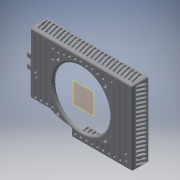
# Autodesk Inventor part: PCB_Cover
Saved by Autodesk Inventor 2019.3 (Build 233278000, 278)
## iProperties
Created: 2020-10-08
Part Number: PCB_Cover
Material: Generisch
Document SubType Name: Modeling
Designer: Nicolas Frick
Density: 1 g/cm^3
Appearance: Vorgabe
Author: Nicolas Frick
Autodesk Inventor part; units mm, degrees
(part 1 of 2)
ref_plane "YZ Plane" through (0, 0, 0) normal (1, 0, 0) x (0, 1, 0)
ref_plane "XZ Plane" through (0, 0, 0) normal (0, 1, 0) x (-1, 0, 0)
ref_plane "XY Plane" through (0, 0, 0) normal (0, 0, 1) x (1, 0, 0)
sketch "Skizze1" plane through (0, 0, 0) normal (0, 0, 1) x (1, 0, 0)
  circle A0 centre (47.5, -25) radius 2.1 construction
  circle A1 centre (-47.5, 25) radius 2.1 construction
  circle A2 centre (47.5, 25) radius 2.1 construction
  circle A3 centre (-47.5, -25) radius 2.1 construction
  circle A4 centre (47.5, -32.5) radius 4 construction
  circle A5 centre (-30, 32.5) radius 4 construction
  circle A6 centre (32, 32.5) radius 4 construction
  circle A7 centre (-47.5, -3) radius 4 construction
  arc A8 (-52.5, -35.5) -> (-50.5, -37.5) centre (-50.5, -35.5) ccw construction
  line L0 (-50.5, -37.5) -> (50.5, -37.5) construction
  arc A9 (50.5, -37.5) -> (52.5, -35.5) centre (50.5, -35.5) ccw construction
  line L1 (52.5, -35.5) -> (52.5, 35.5) construction
  arc A10 (52.5, 35.5) -> (50.5, 37.5) centre (50.5, 35.5) ccw construction
  line L2 (50.5, 37.5) -> (-50.5, 37.5) construction
  arc A11 (-50.5, 37.5) -> (-52.5, 35.5) centre (-50.5, 35.5) ccw construction
  line L3 (-52.5, 35.5) -> (-52.5, -35.5) construction
  line L4 (50, -35) -> (-50, -35)
  line L5 (-50, -35) -> (-50, 35)
  line L6 (-50, 35) -> (50, 35)
  line L7 (50, 35) -> (50, -35)
  line L8 (50, -35) -> (-50, 35) construction
  line L9 (-50, -35) -> (50, 35) construction
  circle A12 centre (0, 0) radius 30
  line L10 (25, -25) -> (-25, -25) construction
  line L11 (-25, -25) -> (-25, 25) construction
  line L12 (-25, 25) -> (25, 25) construction
  line L13 (25, 25) -> (25, -25) construction
  line L14 (25, -25) -> (-25, 25) construction
  line L15 (-25, -25) -> (25, 25) construction
  circle A13 centre (25, -25) radius 2.1
  circle A14 centre (-25, -25) radius 2.1
  circle A15 centre (-25, 25) radius 2.1
  circle A16 centre (25, 25) radius 2.1
  circle A17 centre (47.5, -32.5) radius 1.35
  circle A18 centre (-47.5, -3) radius 1.35
  circle A19 centre (-30, 32.5) radius 1.35
  circle A20 centre (32, 32.5) radius 1.35
  dimension "d0" = 100
  dimension "d1" = 70
  dimension "d2" = 60
  dimension "d3" = 50
  dimension "d4" = 50
  dimension "d5" = 4.2
  dimension "d6" = 4.2
  dimension "d7" = 4.2
  dimension "d8" = 4.2
  dimension "d11" = 2.7
  dimension "d12" = 2.7
  dimension "d13" = 2.7
  dimension "d14" = 2.7
  constraints: 24 end point, 9 centre point, 8 coincident, 4 midpoint, 4 parallel, 2 horizontal, 2 perpendicular
  measures "d0" distance of L5.end L6.end
  measures "d1" distance of L4.end L5.end
  measures "d2" diameter of A12
  measures "d3" distance of L11.end L12.end
  measures "d4" distance of L10.end L11.end
  measures "d5" diameter of A13
  measures "d6" diameter of A14
  measures "d7" diameter of A15
  measures "d8" diameter of A16
  measures "d11" diameter of A17
  measures "d12" diameter of A18
  measures "d13" diameter of A19
  measures "d14" diameter of A20
extrude "Extrusion2" add sketch "Skizze1" along normal blind 2.5
ref_plane "Arbeitsebene3" through (0, 0, 0) normal (0, 0, 1) x (1, 0, 0)
sketch "Skizze3" plane through (0, 0, 0) normal (0, 0, 1) x (1, 0, 0)
  line L0 (-50, 35) -> (50, 35) projected
  line L1 (50, 35) -> (50, -35) projected
  line L2 (50, -35) -> (-50, -35) projected
  line L3 (-50, -35) -> (-50, 35) projected
  line L4 (-52.5, -37.5) -> (52.5, -37.5) projected
  line L5 (52.5, -37.5) -> (52.5, 37.5) projected
  line L6 (52.5, 37.5) -> (-52.5, 37.5) projected
  line L7 (-52.5, 37.5) -> (-52.5, -37.5) projected
  point P0 (0, 0)
extrude "Extrusion4" add sketch "Skizze3" along normal up to surface (2.5 mm away)
sketch "Skizze4" plane through (0, 0, 2.5) normal (0, 0, 1) x (1, 0, 0)
  line L0 (-52.5, -37.5) -> (-9.5, -37.5)
  line L1 (-9.5, -37.5) -> (-9.5, -29.9953)
  line L2 (-32.8176, -24.5) -> (-52.5, -24.5)
  line L3 (-52.5, -24.5) -> (-52.5, -37.5)
  arc A0 (-32.8176, -24.5) -> (-9.5, -29.9953) centre (-10.5668, 17.6958) ccw
  point P0 (0, 0)
  constraints: 8 end point, 2 parallel, 2 point on circle, 1 centre point, 1 horizontal, 1 perpendicular
extrude "Extrusion5" cut sketch "Skizze4" against normal through all
fillet "Rundung1" radius 2 1 edges at (-9.5, -29.9953, 1.25)
sketch "Skizze13" plane through (0, 0, 2.5) normal (0, 0, 1) x (1, 0, 0)
  line L0 (-9.5, -31.9985) -> (-9.5, -37.5) construction
  line L1 (-52.5, -24.5) -> (-32.8176, -24.5) construction
  arc A0 (-32.8176, -24.5) -> (-11.4624, -29.9989) centre (-10.5668, 17.6958) ccw construction
  arc A1 (-9.5, -31.9985) -> (-11.4624, -29.9989) centre (-11.5, -31.9985) ccw construction
  circle A2 centre (0, 0) radius 30 construction
  circle A3 centre (25, 25) radius 2.1 construction
  circle A4 centre (-25, 25) radius 2.1 construction
  circle A5 centre (-25, -25) radius 2.1 construction
  circle A6 centre (25, -25) radius 2.1 construction
  circle A7 centre (32, 32.5) radius 1.35 construction
  circle A8 centre (-30, 32.5) radius 1.35 construction
  circle A9 centre (-47.5, -3) radius 1.35 construction
  circle A10 centre (47.5, -32.5) radius 1.35 construction
  line L2 (52.5, -37.5) -> (52.5, 37.5) projected
  line L3 (-52.5, 37.5) -> (-52.5, -24.5) projected
  line L4 (52.5, -37.5) -> (-9.5, -37.5)
  line L5 (-52.5, -24.5) -> (-52.5, 37.5)
  line L6 (-52.5, 37.5) -> (52.5, 37.5)
  line L7 (52.5, 37.5) -> (52.5, -37.5)
  line L8 (-9.5, -39.5) -> (54.5, -39.5)
  line L9 (54.5, -39.5) -> (54.5, 39.5)
  line L10 (54.5, 39.5) -> (-54.5, 39.5)
  line L11 (-54.5, 39.5) -> (-54.5, -24.5)
  line L12 (52.5, -37.5) -> (-9.5, -37.5) projected
  line L13 (-9.5, -39.5) -> (-9.5, -37.5)
  line L14 (-52.5, -24.5) -> (-54.5, -24.5)
  line L15 (52.5, -37.5) -> (-9.5, -37.5) projected
  line L16 (52.5, 37.5) -> (52.5, -37.5) projected
  line L17 (-52.5, 37.5) -> (52.5, 37.5) projected
  line L18 (-52.5, -24.5) -> (-52.5, 37.5) projected
  dimension "d104" = 2
  constraints: 20 end point, 4 parallel, 3 perpendicular, 2 point on line, 1 horizontal, 1 vertical, 1 other
  measures "d104" distance between parallel lines of L4 L8
extrude "Extrusion15" add sketch "Skizze13" against normal blind 17
sketch "Skizze14" plane through (54.5, -39.5, 2.5) normal (1, 0, 0) x (0, 0, -1)
  line L0 (0, 79) -> (0, 0) construction
  line L1 (0, 0) -> (17, 0) construction
  line L2 (17, 79) -> (17, 0) construction
  line L3 (0, 79) -> (17, 79) construction
  line L4 (2.5, 2) -> (2.5, 77) construction
  line L5 (2.5, 2) -> (17, 2) construction
  line L6 (2.5, 77) -> (17, 77) construction
  line L7 (14.9363, 0.5048) -> (3.5468, 4.0735)
  line L8 (3.5468, 4.0735) -> (4.1448, 5.982)
  line L9 (4.1448, 5.982) -> (15.5343, 2.4133)
  line L10 (15.5343, 2.4133) -> (14.9363, 0.5048)
  line L11 (4.1448, 9.982) -> (15.5343, 6.4133)
  line L12 (15.5343, 6.4133) -> (14.9363, 4.5048)
  line L13 (14.9363, 4.5048) -> (3.5468, 8.0735)
  line L14 (3.5468, 8.0735) -> (4.1448, 9.982)
  line L15 (4.1448, 13.982) -> (15.5343, 10.4133)
  line L16 (15.5343, 10.4133) -> (14.9363, 8.5048)
  line L17 (14.9363, 8.5048) -> (3.5468, 12.0735)
  line L18 (3.5468, 12.0735) -> (4.1448, 13.982)
  line L19 (4.1448, 17.982) -> (15.5343, 14.4133)
  line L20 (15.5343, 14.4133) -> (14.9363, 12.5048)
  line L21 (14.9363, 12.5048) -> (3.5468, 16.0735)
  line L22 (3.5468, 16.0735) -> (4.1448, 17.982)
  line L23 (4.1448, 21.982) -> (15.5343, 18.4133)
  line L24 (15.5343, 18.4133) -> (14.9363, 16.5048)
  line L25 (14.9363, 16.5048) -> (3.5468, 20.0735)
  line L26 (3.5468, 20.0735) -> (4.1448, 21.982)
  line L27 (4.1448, 25.982) -> (15.5343, 22.4133)
  line L28 (15.5343, 22.4133) -> (14.9363, 20.5048)
  line L29 (14.9363, 20.5048) -> (3.5468, 24.0735)
  line L30 (3.5468, 24.0735) -> (4.1448, 25.982)
  line L31 (4.1448, 29.982) -> (15.5343, 26.4133)
  line L32 (15.5343, 26.4133) -> (14.9363, 24.5048)
  line L33 (14.9363, 24.5048) -> (3.5468, 28.0735)
  line L34 (3.5468, 28.0735) -> (4.1448, 29.982)
  line L35 (4.1448, 33.982) -> (15.5343, 30.4133)
  line L36 (15.5343, 30.4133) -> (14.9363, 28.5048)
  line L37 (14.9363, 28.5048) -> (3.5468, 32.0735)
  line L38 (3.5468, 32.0735) -> (4.1448, 33.982)
  line L39 (4.1448, 37.982) -> (15.5343, 34.4133)
  line L40 (15.5343, 34.4133) -> (14.9363, 32.5048)
  line L41 (14.9363, 32.5048) -> (3.5468, 36.0735)
  line L42 (3.5468, 36.0735) -> (4.1448, 37.982)
  line L43 (4.1448, 41.982) -> (15.5343, 38.4133)
  line L44 (15.5343, 38.4133) -> (14.9363, 36.5048)
  line L45 (14.9363, 36.5048) -> (3.5468, 40.0735)
  line L46 (3.5468, 40.0735) -> (4.1448, 41.982)
  line L47 (4.1448, 45.982) -> (15.5343, 42.4133)
  line L48 (15.5343, 42.4133) -> (14.9363, 40.5048)
  line L49 (14.9363, 40.5048) -> (3.5468, 44.0735)
  line L50 (3.5468, 44.0735) -> (4.1448, 45.982)
  line L51 (4.1448, 49.982) -> (15.5343, 46.4133)
  line L52 (15.5343, 46.4133) -> (14.9363, 44.5048)
  line L53 (14.9363, 44.5048) -> (3.5468, 48.0735)
  line L54 (3.5468, 48.0735) -> (4.1448, 49.982)
  line L55 (4.1448, 53.982) -> (15.5343, 50.4133)
  line L56 (15.5343, 50.4133) -> (14.9363, 48.5048)
  line L57 (14.9363, 48.5048) -> (3.5468, 52.0735)
  line L58 (3.5468, 52.0735) -> (4.1448, 53.982)
  line L59 (4.1448, 57.982) -> (15.5343, 54.4133)
  line L60 (15.5343, 54.4133) -> (14.9363, 52.5048)
  line L61 (14.9363, 52.5048) -> (3.5468, 56.0735)
  line L62 (3.5468, 56.0735) -> (4.1448, 57.982)
  line L63 (4.1448, 61.982) -> (15.5343, 58.4133)
  line L64 (15.5343, 58.4133) -> (14.9363, 56.5048)
  line L65 (14.9363, 56.5048) -> (3.5468, 60.0735)
  line L66 (3.5468, 60.0735) -> (4.1448, 61.982)
  line L67 (4.1448, 65.982) -> (15.5343, 62.4133)
  line L68 (15.5343, 62.4133) -> (14.9363, 60.5048)
  line L69 (14.9363, 60.5048) -> (3.5468, 64.0735)
  line L70 (3.5468, 64.0735) -> (4.1448, 65.982)
  line L71 (4.1448, 69.982) -> (15.5343, 66.4133)
  line L72 (15.5343, 66.4133) -> (14.9363, 64.5048)
  line L73 (14.9363, 64.5048) -> (3.5468, 68.0735)
  line L74 (3.5468, 68.0735) -> (4.1448, 69.982)
  line L75 (4.1448, 73.982) -> (15.5343, 70.4133)
  line L76 (15.5343, 70.4133) -> (14.9363, 68.5048)
  line L77 (14.9363, 68.5048) -> (3.5468, 72.0735)
  line L78 (3.5468, 72.0735) -> (4.1448, 73.982)
  line L79 (4.1448, 77.982) -> (15.5343, 74.4133)
  line L80 (15.5343, 74.4133) -> (14.9363, 72.5048)
  line L81 (14.9363, 72.5048) -> (3.5468, 76.0735)
  line L82 (3.5468, 76.0735) -> (4.1448, 77.982)
  line L83 (10.965, 75.845) -> (4.2761, 75.845)
  point P0 (2.5, 39.5)
  dimension "d110" = 4
  constraints: 154 end point, 2 parallel, 2 point on line, 1 perpendicular, 1 vertical, 144 other
  measures "d110" distance of L8.end L11.start
extrude "Extrusion16" cut sketch "Skizze14" against normal through all
sketch "Skizze15" plane through (54.5, -39.5, 2.5) normal (1, 0, 0) x (0, 0, -1)
  line L0 (17.5, 3) -> (2.5, 3) construction
  line L1 (0, 0) -> (17, 0) construction
  line L2 (14.9363, 4.5048) -> (3.5468, 8.0735) construction
  line L3 (3.5468, 8.0735) -> (4.1448, 9.982) construction
  line L4 (4.1448, 9.982) -> (15.5343, 6.4133) construction
  line L5 (15.5343, 6.4133) -> (14.9363, 4.5048) construction
  line L6 (14.9363, 12.5048) -> (3.5468, 16.0735) construction
  line L7 (3.5468, 16.0735) -> (4.1448, 17.982) construction
  line L8 (4.1448, 17.982) -> (15.5343, 14.4133) construction
  line L9 (15.5343, 14.4133) -> (14.9363, 12.5048) construction
  line L10 (14.9363, 20.5048) -> (3.5468, 24.0735) construction
  line L11 (3.5468, 24.0735) -> (4.1448, 25.982) construction
  line L12 (4.1448, 25.982) -> (15.5343, 22.4133) construction
  line L13 (15.5343, 22.4133) -> (14.9363, 20.5048) construction
  line L14 (14.9363, 28.5048) -> (3.5468, 32.0735) construction
  line L15 (3.5468, 32.0735) -> (4.1448, 33.982) construction
  line L16 (4.1448, 33.982) -> (15.5343, 30.4133) construction
  line L17 (15.5343, 30.4133) -> (14.9363, 28.5048) construction
  line L18 (14.9363, 36.5048) -> (3.5468, 40.0735) construction
  line L19 (3.5468, 40.0735) -> (4.1448, 41.982) construction
  line L20 (4.1448, 41.982) -> (15.5343, 38.4133) construction
  line L21 (15.5343, 38.4133) -> (14.9363, 36.5048) construction
  line L22 (14.9363, 44.5048) -> (3.5468, 48.0735) construction
  line L23 (3.5468, 48.0735) -> (4.1448, 49.982) construction
  line L24 (4.1448, 49.982) -> (15.5343, 46.4133) construction
  line L25 (15.5343, 46.4133) -> (14.9363, 44.5048) construction
  line L26 (14.9363, 52.5048) -> (3.5468, 56.0735) construction
  line L27 (3.5468, 56.0735) -> (4.1448, 57.982) construction
  line L28 (4.1448, 57.982) -> (15.5343, 54.4133) construction
  line L29 (15.5343, 54.4133) -> (14.9363, 52.5048) construction
  line L30 (14.9363, 60.5048) -> (3.5468, 64.0735) construction
  line L31 (3.5468, 64.0735) -> (4.1448, 65.982) construction
  line L32 (4.1448, 65.982) -> (15.5343, 62.4133) construction
  line L33 (15.5343, 62.4133) -> (14.9363, 60.5048) construction
  line L34 (14.9363, 68.5048) -> (3.5468, 72.0735) construction
  line L35 (3.5468, 72.0735) -> (4.1448, 73.982) construction
  line L36 (4.1448, 73.982) -> (15.5343, 70.4133) construction
  line L37 (15.5343, 70.4133) -> (14.9363, 68.5048) construction
  line L38 (15.5343, 74.4133) -> (14.9363, 72.5048) construction
  line L39 (14.9363, 72.5048) -> (3.5468, 76.0735) construction
  line L40 (3.5468, 76.0735) -> (4.1448, 77.982) construction
  line L41 (4.1448, 77.982) -> (15.5343, 74.4133) construction
  line L42 (14.9363, 64.5048) -> (3.5468, 68.0735) construction
  line L43 (3.5468, 68.0735) -> (4.1448, 69.982) construction
  line L44 (4.1448, 69.982) -> (15.5343, 66.4133) construction
  line L45 (15.5343, 66.4133) -> (14.9363, 64.5048) construction
  line L46 (14.9363, 56.5048) -> (3.5468, 60.0735) construction
  line L47 (3.5468, 60.0735) -> (4.1448, 61.982) construction
  line L48 (4.1448, 61.982) -> (15.5343, 58.4133) construction
  line L49 (15.5343, 58.4133) -> (14.9363, 56.5048) construction
  line L50 (14.9363, 48.5048) -> (3.5468, 52.0735) construction
  line L51 (3.5468, 52.0735) -> (4.1448, 53.982) construction
  line L52 (4.1448, 53.982) -> (15.5343, 50.4133) construction
  line L53 (15.5343, 50.4133) -> (14.9363, 48.5048) construction
  line L54 (14.9363, 40.5048) -> (3.5468, 44.0735) construction
  line L55 (3.5468, 44.0735) -> (4.1448, 45.982) construction
  line L56 (4.1448, 45.982) -> (15.5343, 42.4133) construction
  line L57 (15.5343, 42.4133) -> (14.9363, 40.5048) construction
  line L58 (14.9363, 32.5048) -> (3.5468, 36.0735) construction
  line L59 (3.5468, 36.0735) -> (4.1448, 37.982) construction
  line L60 (4.1448, 37.982) -> (15.5343, 34.4133) construction
  line L61 (15.5343, 34.4133) -> (14.9363, 32.5048) construction
  line L62 (14.9363, 24.5048) -> (3.5468, 28.0735) construction
  line L63 (3.5468, 28.0735) -> (4.1448, 29.982) construction
  line L64 (4.1448, 29.982) -> (15.5343, 26.4133) construction
  line L65 (15.5343, 26.4133) -> (14.9363, 24.5048) construction
  line L66 (14.9363, 16.5048) -> (3.5468, 20.0735) construction
  line L67 (3.5468, 20.0735) -> (4.1448, 21.982) construction
  line L68 (4.1448, 21.982) -> (15.5343, 18.4133) construction
  line L69 (15.5343, 18.4133) -> (14.9363, 16.5048) construction
  line L70 (14.9363, 8.5048) -> (3.5468, 12.0735) construction
  line L71 (3.5468, 12.0735) -> (4.1448, 13.982) construction
  line L72 (4.1448, 13.982) -> (15.5343, 10.4133) construction
  line L73 (15.5343, 10.4133) -> (14.9363, 8.5048) construction
  line L74 (15.5343, 2.4133) -> (14.9363, 0.5048) construction
  line L75 (14.9363, 0.5048) -> (3.5468, 4.0735) construction
  line L76 (3.5468, 4.0735) -> (4.1448, 5.982) construction
  line L77 (4.1448, 5.982) -> (15.5343, 2.4133) construction
  line L78 (0, 79) -> (0, 0) construction
  line L79 (0, 0) -> (17, 0) construction
  line L80 (17, 79) -> (17, 0) construction
  line L81 (0, 79) -> (17, 79) construction
  line L82 (0, 79) -> (0, 0) construction
  line L83 (7.279, 77) -> (17, 77) construction
  line L84 (14.9363, 0.5048) -> (3.5468, 4.0735) construction
  line L85 (2.5, 2) -> (10.1645, 2) construction
  line L86 (7.279, 2) -> (17, 2)
  line L87 (17, 2) -> (17, 0)
  line L88 (17, 0) -> (7.279, 0)
  line L89 (7.279, 0) -> (7.279, 2)
  point P0 (2.5, 39.5)
  constraints: 10 end point, 2 horizontal, 2 parallel, 2 point on line, 1 perpendicular, 2 other
extrude "Extrusion17" add sketch "Skizze15" against normal up to surface (64 mm away)
sketch "Skizze16" plane through (54.5, -39.5, 2.5) normal (1, 0, 0) x (0, 0, -1)
  line L0 (7.279, 77) -> (17, 77) projected
  line L1 (0, 79) -> (17, 79) projected
  line L2 (17, 77) -> (0, 77)
  line L3 (0, 77) -> (0, 79)
  line L4 (0, 79) -> (17, 79)
  line L5 (17, 79) -> (17, 77)
  point P0 (2.5, 39.5)
  constraints: 8 end point, 2 parallel, 1 horizontal, 1 perpendicular
extrude "Extrusion18" add sketch "Skizze16" against normal up to surface (109 mm away)
sketch "Skizze17" plane through (-54.5, -24.5, 2.5) normal (-1, 0, 0) x (0, 0, 1)
  line L0 (-17, 0) -> (-17, 64) construction
  line L1 (-13.6619, 0) -> (-17, 0) construction
  line L2 (-13.6619, 0) -> (-4.1448, 2.982) construction
  line L3 (-4.1448, 2.982) -> (-3.5468, 1.0735) construction
  line L4 (-3.5468, 1.0735) -> (-6.973, 0) construction
  line L5 (0, 0) -> (-6.973, 0) construction
  line L6 (0, 0) -> (0, 64) construction
  line L7 (0, 64) -> (-17, 64) construction
  line L8 (-3.8371, 62) -> (-7.279, 62) construction
  line L9 (-3.8371, 62) -> (-3.5468, 61.0735) construction
  line L10 (-3.5468, 61.0735) -> (-14.9363, 57.5048) construction
  line L11 (-14.9363, 57.5048) -> (-15.5343, 59.4133) construction
  line L12 (-15.5343, 59.4133) -> (-7.279, 62) construction
  line L13 (-3.5468, 9.0735) -> (-14.9363, 5.5048) construction
  line L14 (-14.9363, 5.5048) -> (-15.5343, 7.4133) construction
  line L15 (-15.5343, 7.4133) -> (-4.1448, 10.982) construction
  line L16 (-4.1448, 10.982) -> (-3.5468, 9.0735) construction
  line L17 (-3.5468, 17.0735) -> (-14.9363, 13.5048) construction
  line L18 (-14.9363, 13.5048) -> (-15.5343, 15.4133) construction
  line L19 (-15.5343, 15.4133) -> (-4.1448, 18.982) construction
  line L20 (-4.1448, 18.982) -> (-3.5468, 17.0735) construction
  line L21 (-3.5468, 25.0735) -> (-14.9363, 21.5048) construction
  line L22 (-14.9363, 21.5048) -> (-15.5343, 23.4133) construction
  line L23 (-15.5343, 23.4133) -> (-4.1448, 26.982) construction
  line L24 (-4.1448, 26.982) -> (-3.5468, 25.0735) construction
  line L25 (-3.5468, 33.0735) -> (-14.9363, 29.5048) construction
  line L26 (-14.9363, 29.5048) -> (-15.5343, 31.4133) construction
  line L27 (-15.5343, 31.4133) -> (-4.1448, 34.982) construction
  line L28 (-4.1448, 34.982) -> (-3.5468, 33.0735) construction
  line L29 (-3.5468, 41.0735) -> (-14.9363, 37.5048) construction
  line L30 (-14.9363, 37.5048) -> (-15.5343, 39.4133) construction
  line L31 (-15.5343, 39.4133) -> (-4.1448, 42.982) construction
  line L32 (-4.1448, 42.982) -> (-3.5468, 41.0735) construction
  line L33 (-3.5468, 49.0735) -> (-14.9363, 45.5048) construction
  line L34 (-14.9363, 45.5048) -> (-15.5343, 47.4133) construction
  line L35 (-15.5343, 47.4133) -> (-4.1448, 50.982) construction
  line L36 (-4.1448, 50.982) -> (-3.5468, 49.0735) construction
  line L37 (-3.5468, 57.0735) -> (-14.9363, 53.5048) construction
  line L38 (-14.9363, 53.5048) -> (-15.5343, 55.4133) construction
  line L39 (-15.5343, 55.4133) -> (-4.1448, 58.982) construction
  line L40 (-4.1448, 58.982) -> (-3.5468, 57.0735) construction
  line L41 (-3.5468, 53.0735) -> (-14.9363, 49.5048) construction
  line L42 (-14.9363, 49.5048) -> (-15.5343, 51.4133) construction
  line L43 (-15.5343, 51.4133) -> (-4.1448, 54.982) construction
  line L44 (-4.1448, 54.982) -> (-3.5468, 53.0735) construction
  line L45 (-3.5468, 45.0735) -> (-14.9363, 41.5048) construction
  line L46 (-14.9363, 41.5048) -> (-15.5343, 43.4133) construction
  line L47 (-15.5343, 43.4133) -> (-4.1448, 46.982) construction
  line L48 (-4.1448, 46.982) -> (-3.5468, 45.0735) construction
  line L49 (-3.5468, 37.0735) -> (-14.9363, 33.5048) construction
  line L50 (-14.9363, 33.5048) -> (-15.5343, 35.4133) construction
  line L51 (-15.5343, 35.4133) -> (-4.1448, 38.982) construction
  line L52 (-4.1448, 38.982) -> (-3.5468, 37.0735) construction
  line L53 (-3.5468, 29.0735) -> (-14.9363, 25.5048) construction
  line L54 (-14.9363, 25.5048) -> (-15.5343, 27.4133) construction
  line L55 (-15.5343, 27.4133) -> (-4.1448, 30.982) construction
  line L56 (-4.1448, 30.982) -> (-3.5468, 29.0735) construction
  line L57 (-3.5468, 21.0735) -> (-14.9363, 17.5048) construction
  line L58 (-14.9363, 17.5048) -> (-15.5343, 19.4133) construction
  line L59 (-15.5343, 19.4133) -> (-4.1448, 22.982) construction
  line L60 (-4.1448, 22.982) -> (-3.5468, 21.0735) construction
  line L61 (-3.5468, 13.0735) -> (-14.9363, 9.5048) construction
  line L62 (-14.9363, 9.5048) -> (-15.5343, 11.4133) construction
  line L63 (-15.5343, 11.4133) -> (-4.1448, 14.982) construction
  line L64 (-4.1448, 14.982) -> (-3.5468, 13.0735) construction
  line L65 (-3.5468, 5.0735) -> (-14.9363, 1.5048) construction
  line L66 (-14.9363, 1.5048) -> (-15.5343, 3.4133) construction
  line L67 (-15.5343, 3.4133) -> (-4.1448, 6.982) construction
  line L68 (-4.1448, 6.982) -> (-3.5468, 5.0735) construction
  line L69 (-17, -13) -> (-17, 62) projected
  line L70 (0, 0) -> (-17, 0)
  line L71 (-17, 0) -> (-17, 1.0735)
  line L72 (-17, 1.0735) -> (0, 1.0735)
  line L73 (0, 1.0735) -> (0, 0)
  point P0 (-2.5, 24.5)
  constraints: 8 end point, 2 parallel, 1 horizontal, 1 perpendicular, 1 point on line
extrude "Extrusion19" add sketch "Skizze17" against normal up to surface (2 mm away)
sketch "Skizze18" plane through (-54.5, 39.5, 2.5) normal (0, 1, 0) x (1, 0, 0)
  line L0 (0, 0) -> (109, 0) construction
  line L1 (109, 0) -> (109, 17) construction
  line L2 (0, 17) -> (109, 17) construction
  line L3 (0, 0) -> (0, 17) construction
  line L4 (107, 2.5) -> (2, 2.5) construction
  line L5 (2, 14.9363) -> (2, 3.5468) construction
  line L6 (107, 7.279) -> (107, 17) construction
  line L7 (101.1704, 15.5042) -> (104.5632, 3.3084)
  line L8 (104.5632, 3.3084) -> (106.49, 3.8445)
  line L9 (106.49, 3.8445) -> (103.0973, 16.0402)
  line L10 (103.0973, 16.0402) -> (101.1704, 15.5042)
  line L11 (97.1704, 15.5042) -> (100.5632, 3.3084)
  line L12 (100.5632, 3.3084) -> (102.49, 3.8445)
  line L13 (102.49, 3.8445) -> (99.0973, 16.0402)
  line L14 (99.0973, 16.0402) -> (97.1704, 15.5042)
  line L15 (93.1704, 15.5042) -> (96.5632, 3.3084)
  line L16 (96.5632, 3.3084) -> (98.49, 3.8445)
  line L17 (98.49, 3.8445) -> (95.0973, 16.0402)
  line L18 (95.0973, 16.0402) -> (93.1704, 15.5042)
  line L19 (89.1704, 15.5042) -> (92.5632, 3.3084)
  line L20 (92.5632, 3.3084) -> (94.49, 3.8445)
  line L21 (94.49, 3.8445) -> (91.0973, 16.0402)
  line L22 (91.0973, 16.0402) -> (89.1704, 15.5042)
  line L23 (85.1704, 15.5042) -> (88.5632, 3.3084)
  line L24 (88.5632, 3.3084) -> (90.49, 3.8445)
  line L25 (90.49, 3.8445) -> (87.0973, 16.0402)
  line L26 (87.0973, 16.0402) -> (85.1704, 15.5042)
  line L27 (81.1704, 15.5042) -> (84.5632, 3.3084)
  line L28 (84.5632, 3.3084) -> (86.49, 3.8445)
  line L29 (86.49, 3.8445) -> (83.0973, 16.0402)
  line L30 (83.0973, 16.0402) -> (81.1704, 15.5042)
  line L31 (77.1704, 15.5042) -> (80.5632, 3.3084)
  line L32 (80.5632, 3.3084) -> (82.49, 3.8445)
  line L33 (82.49, 3.8445) -> (79.0973, 16.0402)
  line L34 (79.0973, 16.0402) -> (77.1704, 15.5042)
  line L35 (73.1704, 15.5042) -> (76.5632, 3.3084)
  line L36 (76.5632, 3.3084) -> (78.49, 3.8445)
  line L37 (78.49, 3.8445) -> (75.0973, 16.0402)
  line L38 (75.0973, 16.0402) -> (73.1704, 15.5042)
  line L39 (69.1704, 15.5042) -> (72.5632, 3.3084)
  line L40 (72.5632, 3.3084) -> (74.49, 3.8445)
  line L41 (74.49, 3.8445) -> (71.0973, 16.0402)
  line L42 (71.0973, 16.0402) -> (69.1704, 15.5042)
  line L43 (65.1704, 15.5042) -> (68.5632, 3.3084)
  line L44 (68.5632, 3.3084) -> (70.49, 3.8445)
  line L45 (70.49, 3.8445) -> (67.0973, 16.0402)
  line L46 (67.0973, 16.0402) -> (65.1704, 15.5042)
  line L47 (61.1704, 15.5042) -> (64.5632, 3.3084)
  line L48 (64.5632, 3.3084) -> (66.49, 3.8445)
  line L49 (66.49, 3.8445) -> (63.0973, 16.0402)
  line L50 (63.0973, 16.0402) -> (61.1704, 15.5042)
  line L51 (57.1704, 15.5042) -> (60.5632, 3.3084)
  line L52 (60.5632, 3.3084) -> (62.49, 3.8445)
  line L53 (62.49, 3.8445) -> (59.0973, 16.0402)
  line L54 (59.0973, 16.0402) -> (57.1704, 15.5042)
  line L55 (53.1704, 15.5042) -> (56.5632, 3.3084)
  line L56 (56.5632, 3.3084) -> (58.49, 3.8445)
  line L57 (58.49, 3.8445) -> (55.0973, 16.0402)
  line L58 (55.0973, 16.0402) -> (53.1704, 15.5042)
  line L59 (49.1704, 15.5042) -> (52.5632, 3.3084)
  line L60 (52.5632, 3.3084) -> (54.49, 3.8445)
  line L61 (54.49, 3.8445) -> (51.0973, 16.0402)
  line L62 (51.0973, 16.0402) -> (49.1704, 15.5042)
  line L63 (45.1704, 15.5042) -> (48.5632, 3.3084)
  line L64 (48.5632, 3.3084) -> (50.49, 3.8445)
  line L65 (50.49, 3.8445) -> (47.0973, 16.0402)
  line L66 (47.0973, 16.0402) -> (45.1704, 15.5042)
  line L67 (41.1704, 15.5042) -> (44.5632, 3.3084)
  line L68 (44.5632, 3.3084) -> (46.49, 3.8445)
  line L69 (46.49, 3.8445) -> (43.0973, 16.0402)
  line L70 (43.0973, 16.0402) -> (41.1704, 15.5042)
  line L71 (37.1704, 15.5042) -> (40.5632, 3.3084)
  line L72 (40.5632, 3.3084) -> (42.49, 3.8445)
  line L73 (42.49, 3.8445) -> (39.0973, 16.0402)
  line L74 (39.0973, 16.0402) -> (37.1704, 15.5042)
  line L75 (33.1704, 15.5042) -> (36.5632, 3.3084)
  line L76 (36.5632, 3.3084) -> (38.49, 3.8445)
  line L77 (38.49, 3.8445) -> (35.0973, 16.0402)
  line L78 (35.0973, 16.0402) -> (33.1704, 15.5042)
  line L79 (29.1704, 15.5042) -> (32.5632, 3.3084)
  line L80 (32.5632, 3.3084) -> (34.49, 3.8445)
  line L81 (34.49, 3.8445) -> (31.0973, 16.0402)
  line L82 (31.0973, 16.0402) -> (29.1704, 15.5042)
  line L83 (25.1704, 15.5042) -> (28.5632, 3.3084)
  line L84 (28.5632, 3.3084) -> (30.49, 3.8445)
  line L85 (30.49, 3.8445) -> (27.0973, 16.0402)
  line L86 (27.0973, 16.0402) -> (25.1704, 15.5042)
  line L87 (21.1704, 15.5042) -> (24.5632, 3.3084)
  line L88 (24.5632, 3.3084) -> (26.49, 3.8445)
  line L89 (26.49, 3.8445) -> (23.0973, 16.0402)
  line L90 (23.0973, 16.0402) -> (21.1704, 15.5042)
  line L91 (17.1704, 15.5042) -> (20.5632, 3.3084)
  line L92 (20.5632, 3.3084) -> (22.49, 3.8445)
  line L93 (22.49, 3.8445) -> (19.0973, 16.0402)
  line L94 (19.0973, 16.0402) -> (17.1704, 15.5042)
  line L95 (13.1704, 15.5042) -> (16.5632, 3.3084)
  line L96 (16.5632, 3.3084) -> (18.49, 3.8445)
  line L97 (18.49, 3.8445) -> (15.0973, 16.0402)
  line L98 (15.0973, 16.0402) -> (13.1704, 15.5042)
  line L99 (9.1704, 15.5042) -> (12.5632, 3.3084)
  line L100 (12.5632, 3.3084) -> (14.49, 3.8445)
  line L101 (14.49, 3.8445) -> (11.0973, 16.0402)
  line L102 (11.0973, 16.0402) -> (9.1704, 15.5042)
  line L103 (5.1704, 15.5042) -> (8.5632, 3.3084)
  line L104 (8.5632, 3.3084) -> (10.49, 3.8445)
  line L105 (10.49, 3.8445) -> (7.0973, 16.0402)
  line L106 (7.0973, 16.0402) -> (5.1704, 15.5042)
  line L107 (1, 18) -> (110, 18) construction
  line L108 (108, 3.5) -> (3, 3.5) construction
  line L109 (3, 15.9363) -> (3, 4.5468) construction
  line L110 (4.9941, 3.083) -> (6.9209, 3.619)
  line L111 (6.9209, 3.619) -> (3.4084, 16.2456)
  line L112 (3.4084, 16.2456) -> (3, 16.132)
  line L113 (3, 10.2511) -> (3, 16.132)
  line L114 (3, 10.2511) -> (4.9941, 3.083)
  point P0 (54.5, 2.5)
  point P1 (103, 2.5)
  point P2 (103, 7.279)
  point P3 (103, 17)
  point P4 (99, 2.5)
  point P5 (99, 7.279)
  point P6 (99, 17)
  point P7 (95, 2.5)
  point P8 (95, 7.279)
  point P9 (95, 17)
  point P10 (91, 2.5)
  point P11 (91, 7.279)
  point P12 (91, 17)
  point P13 (87, 2.5)
  point P14 (87, 7.279)
  point P15 (87, 17)
  point P16 (83, 2.5)
  point P17 (83, 7.279)
  point P18 (83, 17)
  point P19 (79, 2.5)
  point P20 (79, 7.279)
  point P21 (79, 17)
  point P22 (75, 2.5)
  point P23 (75, 7.279)
  point P24 (75, 17)
  point P25 (71, 2.5)
  point P26 (71, 7.279)
  point P27 (71, 17)
  point P28 (67, 2.5)
  point P29 (67, 7.279)
  point P30 (67, 17)
  point P31 (63, 2.5)
  point P32 (63, 7.279)
  point P33 (63, 17)
  point P34 (59, 2.5)
  point P35 (59, 7.279)
  point P36 (59, 17)
  point P37 (55, 2.5)
  point P38 (55, 7.279)
  point P39 (55, 17)
  point P40 (51, 2.5)
  point P41 (51, 7.279)
  point P42 (51, 17)
  point P43 (47, 2.5)
  point P44 (47, 7.279)
  point P45 (47, 17)
  point P46 (43, 2.5)
  point P47 (43, 7.279)
  point P48 (43, 17)
  point P49 (39, 2.5)
  point P50 (39, 7.279)
  point P51 (39, 17)
  point P52 (35, 2.5)
  point P53 (35, 7.279)
  point P54 (35, 17)
  point P55 (31, 2.5)
  point P56 (31, 7.279)
  point P57 (31, 17)
  point P58 (27, 2.5)
  point P59 (27, 7.279)
  point P60 (27, 17)
  point P61 (23, 2.5)
  point P62 (23, 7.279)
  point P63 (23, 17)
  point P64 (19, 2.5)
  point P65 (19, 7.279)
  point P66 (19, 17)
  point P67 (15, 2.5)
  point P68 (15, 7.279)
  point P69 (15, 17)
  point P70 (11, 2.5)
  point P71 (11, 7.279)
  point P72 (11, 17)
  point P73 (55.5, 3.5)
  point P74 (108, 18)
  dimension "d123" = 2
  dimension "d126" = 4
  constraints: 216 end point, 2 parallel, 2 point on line, 1 horizontal, 1 perpendicular, 264 other
  measures "d123" distance of L8.end L7.end
  measures "d126" distance of L4.start point (103, 2.5)
extrude "Extrusion20" cut sketch "Skizze18" against normal through all
sketch "Skizze19" plane through (-9.5, -39.5, 2.5) normal (0, -1, 0) x (1, 0, 0)
  line L0 (0, -3.43) -> (1.49, -3.8445) construction
  line L1 (1.49, -3.8445) -> (0, -9.2005) construction
  line L2 (0, -9.2005) -> (0, -17) construction
  line L3 (64, -17) -> (0, -17) construction
  line L4 (64, 0) -> (64, -17) construction
  line L5 (64, 0) -> (0, 0) construction
  line L6 (0, 0) -> (0, -3.43) construction
  line L7 (59.5632, -3.3084) -> (61.49, -3.8445) construction
  line L8 (61.49, -3.8445) -> (58.0973, -16.0402) construction
  line L9 (58.0973, -16.0402) -> (56.1704, -15.5042) construction
  line L10 (56.1704, -15.5042) -> (59.5632, -3.3084) construction
  line L11 (51.5632, -3.3084) -> (53.49, -3.8445) construction
  line L12 (53.49, -3.8445) -> (50.0973, -16.0402) construction
  line L13 (50.0973, -16.0402) -> (48.1704, -15.5042) construction
  line L14 (48.1704, -15.5042) -> (51.5632, -3.3084) construction
  line L15 (43.5632, -3.3084) -> (45.49, -3.8445) construction
  line L16 (45.49, -3.8445) -> (42.0973, -16.0402) construction
  line L17 (42.0973, -16.0402) -> (40.1704, -15.5042) construction
  line L18 (40.1704, -15.5042) -> (43.5632, -3.3084) construction
  line L19 (35.5632, -3.3084) -> (37.49, -3.8445) construction
  line L20 (37.49, -3.8445) -> (34.0973, -16.0402) construction
  line L21 (34.0973, -16.0402) -> (32.1704, -15.5042) construction
  line L22 (32.1704, -15.5042) -> (35.5632, -3.3084) construction
  line L23 (27.5632, -3.3084) -> (29.49, -3.8445) construction
  line L24 (29.49, -3.8445) -> (26.0973, -16.0402) construction
  line L25 (26.0973, -16.0402) -> (24.1704, -15.5042) construction
  line L26 (24.1704, -15.5042) -> (27.5632, -3.3084) construction
  line L27 (19.5632, -3.3084) -> (21.49, -3.8445) construction
  line L28 (21.49, -3.8445) -> (18.0973, -16.0402) construction
  line L29 (18.0973, -16.0402) -> (16.1704, -15.5042) construction
  line L30 (16.1704, -15.5042) -> (19.5632, -3.3084) construction
  line L31 (11.5632, -3.3084) -> (13.49, -3.8445) construction
  line L32 (13.49, -3.8445) -> (10.0973, -16.0402) construction
  line L33 (10.0973, -16.0402) -> (8.1704, -15.5042) construction
  line L34 (8.1704, -15.5042) -> (11.5632, -3.3084) construction
  line L35 (3.5632, -3.3084) -> (5.49, -3.8445) construction
  line L36 (5.49, -3.8445) -> (2.0973, -16.0402) construction
  line L37 (2.0973, -16.0402) -> (0.1704, -15.5042) construction
  line L38 (0.1704, -15.5042) -> (3.5632, -3.3084) construction
  line L39 (7.5632, -3.3084) -> (9.49, -3.8445) construction
  line L40 (9.49, -3.8445) -> (6.0973, -16.0402) construction
  line L41 (6.0973, -16.0402) -> (4.1704, -15.5042) construction
  line L42 (4.1704, -15.5042) -> (7.5632, -3.3084) construction
  line L43 (15.5632, -3.3084) -> (17.49, -3.8445) construction
  line L44 (17.49, -3.8445) -> (14.0973, -16.0402) construction
  line L45 (14.0973, -16.0402) -> (12.1704, -15.5042) construction
  line L46 (12.1704, -15.5042) -> (15.5632, -3.3084) construction
  line L47 (23.5632, -3.3084) -> (25.49, -3.8445) construction
  line L48 (25.49, -3.8445) -> (22.0973, -16.0402) construction
  line L49 (22.0973, -16.0402) -> (20.1704, -15.5042) construction
  line L50 (20.1704, -15.5042) -> (23.5632, -3.3084) construction
  line L51 (31.5632, -3.3084) -> (33.49, -3.8445) construction
  line L52 (33.49, -3.8445) -> (30.0973, -16.0402) construction
  line L53 (30.0973, -16.0402) -> (28.1704, -15.5042) construction
  line L54 (28.1704, -15.5042) -> (31.5632, -3.3084) construction
  line L55 (39.5632, -3.3084) -> (41.49, -3.8445) construction
  line L56 (41.49, -3.8445) -> (38.0973, -16.0402) construction
  line L57 (38.0973, -16.0402) -> (36.1704, -15.5042) construction
  line L58 (36.1704, -15.5042) -> (39.5632, -3.3084) construction
  line L59 (47.5632, -3.3084) -> (49.49, -3.8445) construction
  line L60 (49.49, -3.8445) -> (46.0973, -16.0402) construction
  line L61 (46.0973, -16.0402) -> (44.1704, -15.5042) construction
  line L62 (44.1704, -15.5042) -> (47.5632, -3.3084) construction
  line L63 (55.5632, -3.3084) -> (57.49, -3.8445) construction
  line L64 (57.49, -3.8445) -> (54.0973, -16.0402) construction
  line L65 (54.0973, -16.0402) -> (52.1704, -15.5042) construction
  line L66 (52.1704, -15.5042) -> (55.5632, -3.3084) construction
  line L67 (0.1704, -15.5042) -> (3.5632, -3.3084) projected
  line L68 (0, 0) -> (1.7177, 0)
  line L69 (1.7177, 0) -> (1.7177, -9.9423)
  line L70 (1.7177, -9.9423) -> (0, -9.9423)
  line L71 (0, -9.9423) -> (0, 0)
  point P0 (9.5, -2.5)
  constraints: 8 end point, 2 parallel, 1 horizontal, 1 perpendicular, 1 point on line
extrude "Extrusion21" add sketch "Skizze19" against normal blind 2
sketch "Skizze20" plane through (0, 0, 2.5) normal (0, 0, 1) x (1, 0, 0)
  circle A0 centre (0, 0) radius 30 construction
  circle A1 centre (25, 25) radius 2.1 construction
  circle A2 centre (-25, 25) radius 2.1 construction
  circle A3 centre (-25, -25) radius 2.1 construction
  circle A4 centre (25, -25) radius 2.1 construction
  circle A5 centre (32, 32.5) radius 1.35 construction
  circle A6 centre (-30, 32.5) radius 1.35 construction
  circle A7 centre (-47.5, -3) radius 1.35 construction
  circle A8 centre (47.5, -32.5) radius 1.35 construction
  line L0 (-9.5, -31.9985) -> (-9.5, -39.5) construction
  line L1 (54.5, -39.5) -> (-9.5, -39.5) construction
  line L2 (54.5, 39.5) -> (54.5, -39.5) construction
  line L3 (-54.5, 39.5) -> (54.5, 39.5) construction
  line L4 (-54.5, -24.5) -> (-54.5, 39.5) construction
  line L5 (-54.5, -24.5) -> (-32.8176, -24.5) construction
  arc A9 (-32.8176, -24.5) -> (-11.4624, -29.9989) centre (-10.5668, 17.6958) ccw construction
  arc A10 (-9.5, -31.9985) -> (-11.4624, -29.9989) centre (-11.5, -31.9985) ccw construction
  line L6 (-52.5, 37.5) -> (-52.5, -24.5) construction
  line L7 (52.5, 37.5) -> (-52.5, 37.5) construction
  line L8 (52.5, -37.5) -> (52.5, 37.5) construction
  line L9 (-9.5, -37.5) -> (52.5, -37.5) construction
  circle A11 centre (47.5, -32.5) radius 4 construction
  circle A12 centre (32, 32.5) radius 4 construction
  circle A13 centre (-30, 32.5) radius 4 construction
  circle A14 centre (-47.5, -3) radius 4 construction
  line L10 (-49.9777, 35.6804) -> (-47.5, 35.6804) construction
  line L11 (-47.5, 35.6804) -> (-47.5, -35.7623) construction
  line L12 (-47.5, -35.7623) -> (-49.9777, -35.7623) construction
  line L13 (-49.9777, -35.7623) -> (-49.9777, 35.6804) construction
  line L14 (-41.5, -35.7623) -> (-43.9777, -35.7623) construction
  line L15 (-41.5, 35.6804) -> (-41.5, -35.7623) construction
  line L16 (-43.9777, -35.7623) -> (-43.9777, 35.6804) construction
  line L17 (-43.9777, 35.6804) -> (-41.5, 35.6804) construction
  line L18 (-35.5, -35.7623) -> (-37.9777, -35.7623) construction
  line L19 (-35.5, 35.6804) -> (-35.5, -35.7623) construction
  line L20 (-37.9777, -35.7623) -> (-37.9777, 35.6804) construction
  line L21 (-37.9777, 35.6804) -> (-35.5, 35.6804) construction
  line L22 (-29.5, -35.7623) -> (-31.9777, -35.7623) construction
  line L23 (-29.5, 35.6804) -> (-29.5, -35.7623) construction
  line L24 (-31.9777, -35.7623) -> (-31.9777, 35.6804) construction
  line L25 (-31.9777, 35.6804) -> (-29.5, 35.6804) construction
  line L26 (-23.5, -35.7623) -> (-25.9777, -35.7623) construction
  line L27 (-23.5, 35.6804) -> (-23.5, -35.7623) construction
  line L28 (-25.9777, -35.7623) -> (-25.9777, 35.6804) construction
  line L29 (-25.9777, 35.6804) -> (-23.5, 35.6804) construction
  line L30 (-17.5, -35.7623) -> (-19.9777, -35.7623) construction
  line L31 (-17.5, 35.6804) -> (-17.5, -35.7623) construction
  line L32 (-19.9777, -35.7623) -> (-19.9777, 35.6804) construction
  line L33 (-19.9777, 35.6804) -> (-17.5, 35.6804) construction
  line L34 (-11.5, -35.7623) -> (-13.9777, -35.7623) construction
  line L35 (-11.5, 35.6804) -> (-11.5, -35.7623) construction
  line L36 (-13.9777, -35.7623) -> (-13.9777, 35.6804) construction
  line L37 (-13.9777, 35.6804) -> (-11.5, 35.6804) construction
  line L38 (-5.5, -35.7623) -> (-7.9777, -35.7623) construction
  line L39 (-5.5, 35.6804) -> (-5.5, -35.7623) construction
  line L40 (-7.9777, -35.7623) -> (-7.9777, 35.6804) construction
  line L41 (-7.9777, 35.6804) -> (-5.5, 35.6804) construction
  line L42 (0.5, -35.7623) -> (-1.9777, -35.7623) construction
  line L43 (0.5, 35.6804) -> (0.5, -35.7623) construction
  line L44 (-1.9777, -35.7623) -> (-1.9777, 35.6804) construction
  line L45 (-1.9777, 35.6804) -> (0.5, 35.6804) construction
  line L46 (6.5, -35.7623) -> (4.0223, -35.7623) construction
  line L47 (6.5, 35.6804) -> (6.5, -35.7623) construction
  line L48 (4.0223, -35.7623) -> (4.0223, 35.6804) construction
  line L49 (4.0223, 35.6804) -> (6.5, 35.6804) construction
  line L50 (12.5, -35.7623) -> (10.0223, -35.7623) construction
  line L51 (12.5, 35.6804) -> (12.5, -35.7623) construction
  line L52 (10.0223, -35.7623) -> (10.0223, 35.6804) construction
  line L53 (10.0223, 35.6804) -> (12.5, 35.6804) construction
  line L54 (18.5, -35.7623) -> (16.0223, -35.7623) construction
  line L55 (18.5, 35.6804) -> (18.5, -35.7623) construction
  line L56 (16.0223, -35.7623) -> (16.0223, 35.6804) construction
  line L57 (16.0223, 35.6804) -> (18.5, 35.6804) construction
  line L58 (24.5, -35.7623) -> (22.0223, -35.7623) construction
  line L59 (24.5, 35.6804) -> (24.5, -35.7623) construction
  line L60 (22.0223, -35.7623) -> (22.0223, 35.6804) construction
  line L61 (22.0223, 35.6804) -> (24.5, 35.6804) construction
  line L62 (30.5, -35.7623) -> (28.0223, -35.7623) construction
  line L63 (30.5, 35.6804) -> (30.5, -35.7623) construction
  line L64 (28.0223, -35.7623) -> (28.0223, 35.6804) construction
  line L65 (28.0223, 35.6804) -> (30.5, 35.6804) construction
  line L66 (36.5, -35.7623) -> (34.0223, -35.7623) construction
  line L67 (36.5, 35.6804) -> (36.5, -35.7623) construction
  line L68 (34.0223, -35.7623) -> (34.0223, 35.6804) construction
  line L69 (34.0223, 35.6804) -> (36.5, 35.6804) construction
  line L70 (42.5, -35.7623) -> (40.0223, -35.7623) construction
  line L71 (42.5, 35.6804) -> (42.5, -35.7623) construction
  line L72 (40.0223, -35.7623) -> (40.0223, 35.6804) construction
  line L73 (40.0223, 35.6804) -> (42.5, 35.6804) construction
  line L74 (48.5, -35.7623) -> (46.0223, -35.7623) construction
  line L75 (48.5, 35.6804) -> (48.5, -35.7623) construction
  line L76 (46.0223, -35.7623) -> (46.0223, 35.6804) construction
  line L77 (46.0223, 35.6804) -> (48.5, 35.6804) construction
  line L78 (-49.9777, -22.9) -> (-29.5, -22.9) construction
  circle A15 centre (0, 0) radius 38.2063 construction
  line L79 (46.0223, 35.6804) -> (48.5, 35.6804)
  line L80 (48.5, 35.6804) -> (48.5, -27.1)
  line L81 (48.5, -27.1) -> (46.0223, -27.1)
  line L82 (46.0223, -27.1) -> (46.0223, 35.6804)
  line L83 (40.0223, 35.6804) -> (42.5, 35.6804)
  line L84 (42.5, 35.6804) -> (42.5, -35.7623)
  line L85 (42.5, -35.7623) -> (40.0223, -35.7623)
  line L86 (40.0223, -35.7623) -> (40.0223, 35.6804)
  line L87 (36.5, -35.7623) -> (34.0223, -35.7623)
  line L88 (34.0223, -35.7623) -> (34.0223, 27.1)
  line L89 (34.0223, 27.1) -> (36.5, 27.1)
  line L90 (36.5, 27.1) -> (36.5, -35.7623)
  line L91 (30.5, -35.7623) -> (28.0223, -35.7623)
  line L92 (28.0223, -35.7623) -> (28.0223, -25.9706)
  line L93 (28.0223, -25.9706) -> (30.5, -25.9706)
  line L94 (30.5, -25.9706) -> (30.5, -35.7623)
  line L95 (24.5, 35.6804) -> (22.0223, 35.6804)
  line L96 (22.0223, 35.6804) -> (22.0223, 30)
  line L97 (22.0223, 30) -> (24.5, 30)
  line L98 (24.5, 30) -> (24.5, 35.6804)
  line L99 (18.5, 35.6804) -> (16.0223, 35.6804)
  line L100 (16.0223, 35.6804) -> (16.0223, 31.6466)
  line L101 (16.0223, 31.6466) -> (18.5, 31.6466)
  line L102 (18.5, 31.6466) -> (18.5, 35.6804)
  line L103 (-19.9777, 35.6804) -> (-17.5, 35.6804)
  line L104 (-17.5, 35.6804) -> (-17.5, 31.3064)
  line L105 (-17.5, 31.3064) -> (-19.9777, 31.3064)
  line L106 (-19.9777, 31.3064) -> (-19.9777, 35.6804)
  line L107 (-25.9777, 35.6804) -> (-23.5, 35.6804)
  line L108 (-23.5, 35.6804) -> (-23.5, 30.1243)
  line L109 (-23.5, 30.1243) -> (-25.9777, 30.1243)
  line L110 (-25.9777, 30.1243) -> (-25.9777, 35.6804)
  line L111 (-37.9777, 35.6804) -> (-35.5, 35.6804)
  line L112 (-35.5, 35.6804) -> (-35.5, -22.9)
  line L113 (-35.5, -22.9) -> (-37.9777, -22.9)
  line L114 (-37.9777, -22.9) -> (-37.9777, 35.6804)
  line L115 (-41.5, -22.9) -> (-43.9777, -22.9)
  line L116 (-43.9777, -22.9) -> (-43.9777, 35.6804)
  line L117 (-43.9777, 35.6804) -> (-41.5, 35.6804)
  line L118 (-41.5, 35.6804) -> (-41.5, -22.9)
  line L119 (-47.5, 35.6804) -> (-49.9777, 35.6804)
  line L120 (-49.9777, 35.6804) -> (-49.9777, -0.041)
  line L121 (-49.9777, -0.041) -> (-47.5, -0.041)
  line L122 (-47.5, -0.041) -> (-47.5, 35.6804)
  line L123 (-49.9777, -6.1402) -> (-47.5, -6.1402)
  line L124 (-47.5, -6.1402) -> (-47.5, -22.9)
  line L125 (-47.5, -22.9) -> (-49.9777, -22.9)
  line L126 (-49.9777, -22.9) -> (-49.9777, -6.1402)
  line L127 (-31.9777, 20.9081) -> (-29.5, 20.9081)
  line L128 (-29.5, 20.9081) -> (-29.5, 27.1)
  line L129 (-29.5, 27.1) -> (-31.9777, 27.1)
  line L130 (-31.9777, 27.1) -> (-31.9777, 20.9081)
  line L131 (-31.9777, -22.9) -> (-29.5, -22.9)
  line L132 (-29.5, -22.9) -> (-29.5, -16.7561)
  line L133 (-29.5, -16.7561) -> (-31.9777, -16.7561)
  line L134 (-31.9777, -16.7561) -> (-31.9777, -22.9)
  line L135 (24.5, -35.7623) -> (22.0223, -35.7623)
  line L136 (22.0223, -35.7623) -> (22.0223, -28.5)
  line L137 (22.0223, -28.5) -> (24.5, -28.5)
  line L138 (24.5, -28.5) -> (24.5, -35.7623)
  line L139 (18.5, -35.7623) -> (16.0223, -35.7623)
  line L140 (16.0223, -35.7623) -> (16.0223, -28.5)
  line L141 (16.0223, -28.5) -> (18.5, -28.5)
  line L142 (18.5, -28.5) -> (18.5, -35.7623)
  line L143 (12.5, -35.7623) -> (10.0223, -35.7623)
  line L144 (10.0223, -35.7623) -> (10.0223, -32.1312)
  line L145 (10.0223, -32.1312) -> (12.5, -32.1312)
  line L146 (12.5, -32.1312) -> (12.5, -35.7623)
  line L147 (6.5, -35.7623) -> (4.0223, -35.7623)
  line L148 (4.0223, -35.7623) -> (4.0223, -33.9467)
  line L149 (4.0223, -33.9467) -> (6.5, -33.9467)
  line L150 (6.5, -33.9467) -> (6.5, -35.7623)
  line L151 (0.5, -35.7623) -> (-1.9777, -35.7623)
  line L152 (-1.9777, -35.7623) -> (-1.9777, -33.9467)
  line L153 (-1.9777, -33.9467) -> (0.5, -33.9467)
  line L154 (0.5, -33.9467) -> (0.5, -35.7623)
  line L155 (-5.5, -35.7623) -> (-7.9777, -35.7623)
  line L156 (-7.9777, -35.7623) -> (-7.9777, -32.1312)
  line L157 (-7.9777, -32.1312) -> (-5.5, -32.1312)
  line L158 (-5.5, -32.1312) -> (-5.5, -35.7623)
  line L159 (-13.9777, 35.6804) -> (-11.5, 35.6804)
  line L160 (-11.5, 35.6804) -> (-11.5, 32.5)
  line L161 (-11.5, 32.5) -> (-13.9777, 32.5)
  line L162 (-13.9777, 32.5) -> (-13.9777, 35.6804)
  line L163 (-7.9777, 35.6804) -> (-5.5, 35.6804)
  line L164 (-5.5, 35.6804) -> (-5.5, 33.0955)
  line L165 (-5.5, 33.0955) -> (-7.9777, 33.0955)
  line L166 (-7.9777, 33.0955) -> (-7.9777, 35.6804)
  line L167 (10.0223, 35.6804) -> (12.5, 35.6804)
  line L168 (12.5, 35.6804) -> (12.5, 32.8979)
  line L169 (12.5, 32.8979) -> (10.0223, 32.8979)
  line L170 (10.0223, 32.8979) -> (10.0223, 35.6804)
  line L171 (4.0223, 35.6804) -> (6.5, 35.6804)
  line L172 (6.5, 35.6804) -> (6.5, 32.8979)
  line L173 (6.5, 32.8979) -> (4.0223, 32.8979)
  line L174 (4.0223, 32.8979) -> (4.0223, 35.6804)
  line L175 (-1.9777, 35.6804) -> (0.5, 35.6804)
  line L176 (0.5, 35.6804) -> (0.5, 34.0902)
  line L177 (0.5, 34.0902) -> (-1.9777, 34.0902)
  line L178 (-1.9777, 34.0902) -> (-1.9777, 35.6804)
  point P0 (-48.5, -24.5)
  point P1 (-48.5, 39.5)
  point P2 (-41.5, -3)
  point P3 (-41.5, -3)
  point P4 (-46.5, -24.5)
  point P5 (-46.5, 37.5)
  point P6 (-42.5, -24.5)
  point P7 (-42.5, 39.5)
  point P8 (-35.5, -3)
  point P9 (-35.5, -3)
  point P10 (-40.5, -24.5)
  point P11 (-40.5, 37.5)
  point P12 (-36.5, -24.5)
  point P13 (-36.5, 39.5)
  point P14 (-29.5, -3)
  point P15 (-29.5, -3)
  point P16 (-34.5, -24.5)
  point P17 (-34.5, 37.5)
  point P18 (-30.5, -24.5)
  point P19 (-30.5, 39.5)
  point P20 (-23.5, -3)
  point P21 (-23.5, -3)
  point P22 (-28.5, -24.5)
  point P23 (-28.5, 37.5)
  point P24 (-24.5, -24.5)
  point P25 (-24.5, 39.5)
  point P26 (-17.5, -3)
  point P27 (-17.5, -3)
  point P28 (-22.5, -24.5)
  point P29 (-22.5, 37.5)
  point P30 (-18.5, -24.5)
  point P31 (-18.5, 39.5)
  point P32 (-11.5, -3)
  point P33 (-11.5, -3)
  point P34 (-16.5, -24.5)
  point P35 (-16.5, 37.5)
  point P36 (-12.5, -24.5)
  point P37 (-12.5, 39.5)
  point P38 (-5.5, -3)
  point P39 (-5.5, -3)
  point P40 (-10.5, -24.5)
  point P41 (-10.5, 37.5)
  point P42 (-6.5, -24.5)
  point P43 (-6.5, 39.5)
  point P44 (0.5, -3)
  point P45 (0.5, -3)
  point P46 (-4.5, -24.5)
  point P47 (-4.5, 37.5)
  point P48 (-0.5, -24.5)
  point P49 (-0.5, 39.5)
  point P50 (6.5, -3)
  point P51 (6.5, -3)
  point P52 (1.5, -24.5)
  point P53 (1.5, 37.5)
  point P54 (5.5, -24.5)
  point P55 (5.5, 39.5)
  point P56 (12.5, -3)
  point P57 (12.5, -3)
  point P58 (7.5, -24.5)
  point P59 (7.5, 37.5)
  point P60 (11.5, -24.5)
  point P61 (11.5, 39.5)
  point P62 (18.5, -3)
  point P63 (18.5, -3)
  point P64 (13.5, -24.5)
  point P65 (13.5, 37.5)
  point P66 (17.5, -24.5)
  point P67 (17.5, 39.5)
  point P68 (24.5, -3)
  point P69 (24.5, -3)
  point P70 (19.5, -24.5)
  point P71 (19.5, 37.5)
  point P72 (23.5, -24.5)
  point P73 (23.5, 39.5)
  point P74 (30.5, -3)
  point P75 (30.5, -3)
  point P76 (25.5, -24.5)
  point P77 (25.5, 37.5)
  point P78 (29.5, -24.5)
  point P79 (29.5, 39.5)
  point P80 (36.5, -3)
  point P81 (36.5, -3)
  point P82 (31.5, -24.5)
  point P83 (31.5, 37.5)
  point P84 (35.5, -24.5)
  point P85 (35.5, 39.5)
  point P86 (42.5, -3)
  point P87 (42.5, -3)
  point P88 (37.5, -24.5)
  point P89 (37.5, 37.5)
  point P90 (41.5, -24.5)
  point P91 (41.5, 39.5)
  point P92 (48.5, -3)
  point P93 (48.5, -3)
  point P94 (43.5, -24.5)
  point P95 (43.5, 37.5)
  dimension "d137" = 6
  constraints: 338 end point, 52 parallel, 37 point on line, 27 horizontal, 27 perpendicular, 3 point on circle, 1 centre point, 1 coincident, 1 midpoint, 226 other
  measures "d137" distance of L4.start point (-48.5, -24.5)
extrude "Extrusion23" cut sketch "Skizze20" against normal blind 2